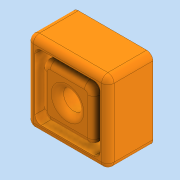
# Autodesk Inventor part: 2_Connettore_inf_sup
Saved by Autodesk Inventor 2020 (Build 240168000, 168)
## iProperties
Created: 2019-10-11
Part Number: 2_Connettore_inf_sup
Material: Generico
Document SubType Name: Modeling
Designer: socci
Density: 1 g/cm^3
Appearance: Arancione
Mass: 37.2193 g
Surface Area: 104.888 cm^2
Volume: 37.2193 cm^3
Author: socci
Autodesk Inventor part; units mm, degrees
ref_plane "YZ Plane" through (0, 0, 0) normal (1, 0, 0) x (0, 1, 0)
ref_plane "XZ Plane" through (0, 0, 0) normal (0, 1, 0) x (-1, 0, 0)
ref_plane "XY Plane" through (0, 0, 0) normal (0, 0, 1) x (1, 0, 0)
sketch "Schizzo1" plane through (0, 0, 0) normal (0, 0, 1) x (1, 0, 0)
  line L0 (6.5, -8.5) -> (-5.5, -8.5)
  line L1 (-8.5, -5.5) -> (-8.5, 5.5)
  line L2 (-5.5, 8.5) -> (5.5, 8.5)
  line L3 (8.5, 5.5) -> (8.5, -6.5)
  arc A0 (6.5, -8.5) -> (8.5, -6.5) centre (6.5, -6.5) ccw
  arc A1 (-8.5, -5.5) -> (-5.5, -8.5) centre (-5.5, -5.5) ccw
  arc A2 (-5.5, 8.5) -> (-8.5, 5.5) centre (-5.5, 5.5) ccw
  arc A3 (8.5, 5.5) -> (5.5, 8.5) centre (5.5, 5.5) ccw
  point P0 (0, 0)
  point P1 (0, 0)
  point P2 (8.5, -8.5)
  point P3 (-8.5, -8.5)
  point P4 (-8.5, 8.5)
  point P5 (8.5, 8.5)
  dimension "d0" = 17
  dimension "d44" = 2
  dimension "d45" = 3
  constraints: 8 end point, 8 point on circle, 8 point on line, 8 tangent, 4 centre point, 2 equal radius, 1 coincident, 9 other
  measures "d0" distance of point (-8.5, 8.5) point (8.5, 8.5)
  measures "d44" radius of A0
  measures "d45" radius of A1
extrude "Estrusione1" add sketch "Schizzo1" along normal blind 10
sketch "Schizzo2" plane through (0, 0, 0) normal (0, 0, -1) x (-1, 0, 0)
  line L0 (11, -13) -> (-11, -13)
  line L1 (-13, -11) -> (-13, 11)
  line L2 (-11, 13) -> (11, 13)
  line L3 (13, 11) -> (13, -11)
  line L4 (13, -13) -> (-13, 13) construction
  line L5 (-13, -13) -> (13, 13) construction
  arc A0 (13, 11) -> (11, 13) centre (11, 11) ccw
  arc A1 (11, -13) -> (13, -11) centre (11, -11) ccw
  arc A2 (-13, -11) -> (-11, -13) centre (-11, -11) ccw
  arc A3 (-11, 13) -> (-13, 11) centre (-11, 11) ccw
  point P0 (0, 0)
  dimension "d3" = 26
  dimension "d4" = 26
  dimension "d145" = 2
  constraints: 12 end point, 8 point on circle, 8 point on line, 8 tangent, 4 centre point, 3 equal radius, 3 midpoint, 2 parallel, 1 horizontal, 1 perpendicular
  measures "d3" distance of L4.start L5.start
  measures "d4" distance of L5.start L4.end
  measures "d145" radius of A0
extrude "Estrusione2" add sketch "Schizzo2" along normal blind 4.5
sketch "Schizzo12" plane through (0, 0, 0) normal (0, 0, 1) x (1, 0, 0)
  line L0 (-10.5, -8.5) -> (-10.5, 8.5)
  line L1 (-8.5, 10.5) -> (8.5, 10.5)
  line L2 (10.5, 8.5) -> (10.5, -8.5)
  line L3 (8.5, -10.5) -> (-8.5, -10.5)
  line L4 (-13, -11) -> (-13, 11)
  line L5 (-11, 13) -> (11, 13)
  line L6 (13, 11) -> (13, -11)
  line L7 (11, -13) -> (-11, -13)
  arc A0 (10.5, 8.5) -> (8.5, 10.5) centre (8.5, 8.5) ccw
  arc A1 (13, 11) -> (11, 13) centre (11, 11) ccw
  arc A2 (11, -13) -> (13, -11) centre (11, -11) ccw
  arc A3 (8.5, -10.5) -> (10.5, -8.5) centre (8.5, -8.5) ccw
  arc A4 (-13, -11) -> (-11, -13) centre (-11, -11) ccw
  arc A5 (-10.5, -8.5) -> (-8.5, -10.5) centre (-8.5, -8.5) ccw
  arc A6 (-11, 13) -> (-13, 11) centre (-11, 11) ccw
  arc A7 (-8.5, 10.5) -> (-10.5, 8.5) centre (-8.5, 8.5) ccw
  point P0 (0, 0)
  point P1 (0, 0)
  point P2 (-10.5, -10.5)
  point P3 (-10.5, 10.5)
  point P4 (10.5, 10.5)
  point P5 (10.5, -10.5)
  point P6 (0, 0)
  point P7 (-13, -13)
  point P8 (-13, 13)
  point P9 (13, 13)
  point P10 (13, -13)
  dimension "d110" = 21
  dimension "d111" = 26
  dimension "d112" = 2
  constraints: 16 end point, 16 point on circle, 16 point on line, 16 tangent, 8 centre point, 7 equal radius, 2 coincident, 18 other
  measures "d110" distance of point (10.5, -10.5) point (-10.5, -10.5)
  measures "d111" distance of point (13, -13) point (-13, -13)
  measures "d112" radius of A0
extrude "Estrusione6" add sketch "Schizzo12" along normal blind 10
fillet "Raccordo3" radius 2 1 edges at (0, -13, 10)
fillet "Raccordo8" radius 2 1 edges at (0, 8.5, 10)
sketch "Schizzo20" plane through (0, 0, 10) normal (0, 0, 1) x (1, 0, 0)
  circle A0 centre (0, 0) radius 3.25
  dimension "d176" = 6.5
  constraints: 1 centre point, 1 coincident
  measures "d176" diameter of A0
extrude "Estrusione9" cut sketch "Schizzo20" against normal blind 10
fillet "Raccordo9" radius 2 1 edges at (-3.25, 0, 10)
sketch "Schizzo21" plane through (0, 0, -4.5) normal (0, 0, -1) x (-1, 0, 0)
  circle A0 centre (0, 0) radius 4
  line L0 (-4, 2.3094) -> (0, 4.6188)
  line L1 (0, 4.6188) -> (4, 2.3094)
  line L2 (4, 2.3094) -> (4, -2.3094)
  line L3 (4, -2.3094) -> (0, -4.6188)
  line L4 (0, -4.6188) -> (-4, -2.3094)
  line L5 (-4, -2.3094) -> (-4, 2.3094)
  point P0 (-4, 0)
  dimension "d180" = 8
  constraints: 12 end point, 2 coincident, 1 horizontal alignment, 1 midpoint, 15 other
extrude "Estrusione10" cut sketch "Schizzo21" against normal blind 2
